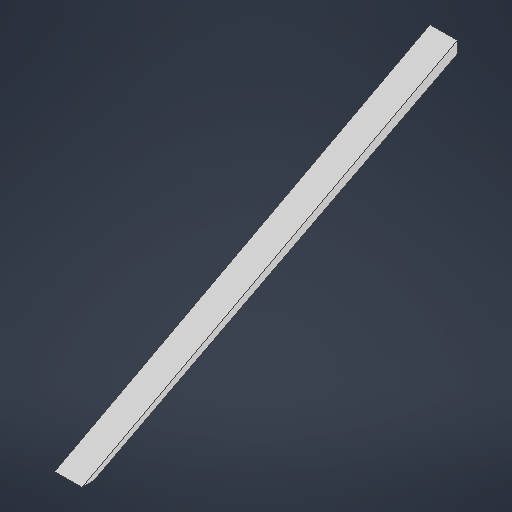
# Autodesk Inventor part: S_2x4x54.35
Saved by Autodesk Inventor 2027.1 (Build 311270010, 270A)
## iProperties
Created: 2026-08-30
Part Number: S_2x4x54.35
Material: Generic
Document SubType Name: Modeling
Designer: jorda
Density: 1 g/cm^3
Appearance: Default
Author: jorda
Autodesk Inventor part; units mm, degrees
ref_plane "YZ Plane" through (0, 0, 0) normal (1, 0, 0) x (0, 1, 0)
ref_plane "XZ Plane" through (0, 0, 0) normal (0, 1, 0) x (-1, 0, 0)
ref_plane "XY Plane" through (0, 0, 0) normal (0, 0, 1) x (1, 0, 0)
sketch "Sketch1" plane through (0, 0, 0) normal (1, 0, 0) x (0, 1, 0)
  line L0 (0, 0) -> (0, -38.1)
  line L1 (647.7, -1219.2) -> (609.6, -1219.2)
  line L2 (609.6, -1219.2) -> (0, -38.1)
  line L3 (0, 0) -> (647.7, -1219.2)
  constraints: 8 end point
extrude "Extrusion1" add sketch "Sketch1" along normal blind 88.9
body "Solid1"
